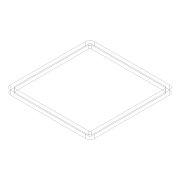
# Autodesk Inventor part: Adult fly trap middle
Saved by Autodesk Inventor 2020 (Build 240168000, 168)
## iProperties
Created: 2020-09-12
Part Number: Adult fly trap middle
Material: Generic
Document SubType Name: Modeling
Designer: ferrerx
Density: 1 g/cm^3
Appearance: Clear - Light
Author: ferrerx
Autodesk Inventor part; units mm, degrees
ref_plane "YZ Plane" through (0, 0, 0) normal (1, 0, 0) x (0, 1, 0)
ref_plane "XZ Plane" through (0, 0, 0) normal (0, 1, 0) x (-1, 0, 0)
ref_plane "XY Plane" through (0, 0, 0) normal (0, 0, 1) x (1, 0, 0)
sketch "Sketch1" plane through (0, 0, 0) normal (0, 1, 0) x (-1, 0, 0)
  line L0 (0, 0) -> (94, 0)
  line L1 (94, 0) -> (94, -94)
  line L2 (94, -94) -> (0, -94)
  line L3 (0, -94) -> (0, 0)
  dimension "d0" = 94
  dimension "d1" = 94
  constraints: 8 end point, 2 parallel, 1 horizontal, 1 perpendicular
  measures "d0" distance of L1.end L2.end
  measures "d1" distance of L2.end L0.start
extrude "Extrusion1" add sketch "Sketch1" along normal blind 5
sketch "Sketch2" plane through (0, 5, 0) normal (0, 1, 0) x (1, 0, 0)
  line L0 (-90, 4) -> (-4, 4)
  line L1 (-4, 4) -> (-4, 90)
  line L2 (-4, 90) -> (-90, 90)
  line L3 (-90, 90) -> (-90, 4)
  line L4 (0, 94) -> (-94, 94) projected
  line L5 (-94, 94) -> (-94, 0) projected
  line L6 (-94, 0) -> (0, 0) projected
  line L7 (0, 0) -> (0, 94) projected
  dimension "d4" = 4
  dimension "d5" = 4
  dimension "d6" = 4
  dimension "d7" = 4
  constraints: 8 end point, 2 parallel, 1 horizontal, 1 perpendicular
  measures "d4" distance between parallel lines of L4 L2
  measures "d5" distance between parallel lines of L5 L3
  measures "d6" distance between parallel lines of L6 L0
  measures "d7" distance between parallel lines of L7 L1
extrude "Extrusion2" cut sketch "Sketch2" against normal blind 5 contours L3 L2 L1 L0
fillet "Fillet1" radius 5 4 edges at (-94, 2.5, -94) (0, 2.5, 0) (0, 2.5, -94) (-94, 2.5, 0)
sketch "Sketch3" plane through (0, 5, 0) normal (0, 1, 0) x (1, 0, 0)
  line L0 (-91.5, 91.5) -> (-2.5, 91.5) construction
  line L1 (-2.5, 91.5) -> (-2.5, 2.5) construction
  line L2 (-2.5, 2.5) -> (-91.5, 2.5) construction
  line L3 (-91.5, 2.5) -> (-91.5, 91.5) construction
  line L4 (0, 5) -> (0, 89) projected
  line L5 (-5, 94) -> (-89, 94) projected
  line L6 (-94, 89) -> (-94, 5) projected
  line L7 (-89, 0) -> (-5, 0) projected
  point P0 (0, 0)
  dimension "d11" = 2.5
  dimension "d12" = 2.5
  dimension "d13" = 2.5
  dimension "d14" = 2.5
  constraints: 8 end point, 2 parallel, 1 horizontal, 1 perpendicular
  measures "d11" distance between parallel lines of L4 L1
  measures "d12" distance between parallel lines of L5 L0
  measures "d13" distance between parallel lines of L6 L3
  measures "d14" distance between parallel lines of L7 L2
fillet "Fillet2" radius 2 4 edges at (-90, 2.5, -90) (-4, 2.5, -90) (-4, 2.5, -4) (-90, 2.5, -4)
body "Solid1"
